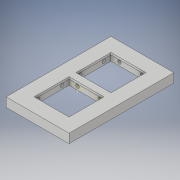
# Autodesk Inventor part: top_plate
Saved by Autodesk Inventor 2018 (Build 220112000, 112)
## iProperties
Created: 2017-12-20
Part Number: top_plate
Material: Generic
Document SubType Name: Modeling
Designer: gaffo
Density: 1 g/cm^3
Appearance: Default
Author: gaffo
Autodesk Inventor part; units mm, degrees
note: some values were not read from the file. Chosen so that the rebuilt part matches the saved one: direction of "Hole6".
ref_plane "YZ Plane" through (0, 0, 0) normal (1, 0, 0) x (0, 1, 0)
ref_plane "XZ Plane" through (0, 0, 0) normal (0, 1, 0) x (-1, 0, 0)
ref_plane "XY Plane" through (0, 0, 0) normal (0, 0, 1) x (1, 0, 0)
sketch "Sketch8" plane through (0, 0, 0) normal (0, 1, 0) x (-1, 0, 0)
  line L0 (45, -75) -> (45, 75) projected
  line L1 (45, 75) -> (-45, 75) projected
  line L2 (-45, 75) -> (-45, -75) projected
  line L3 (-45, -75) -> (45, -75) projected
  line L4 (-27.286, -57.286) -> (-27.286, -2.714) projected
  line L5 (27.286, -57.286) -> (-27.286, -57.286) projected
  line L6 (27.286, -2.714) -> (27.286, -57.286) projected
  line L7 (-27.286, -2.714) -> (27.286, -2.714) projected
  line L8 (27.286, 57.286) -> (27.286, 2.714) projected
  line L9 (27.286, 2.714) -> (-27.286, 2.714) projected
  line L10 (-27.286, 57.286) -> (27.286, 57.286) projected
  line L11 (-27.286, 2.714) -> (-27.286, 57.286) projected
  point P0 (0, 0)
extrude "Extrusion7" add sketch "Sketch8" against normal blind 10
sketch "Sketch2" plane through (0, 0, 0) normal (0, 1, 0) x (-1, 0, 0)
  line L0 (45, 75) -> (-45, 75)
  line L1 (-45, -75) -> (45, -75)
  line L2 (45, -75) -> (45, 75)
  line L3 (-45, 75) -> (-45, -75)
  line L4 (-25, -55) -> (25, -55)
  line L5 (25, -55) -> (25, -5)
  line L6 (25, -5) -> (-25, -5)
  line L7 (-25, -5) -> (-25, -55)
  line L8 (-25, 5) -> (25, 5)
  line L9 (25, 5) -> (25, 55)
  line L10 (25, 55) -> (-25, 55)
  line L11 (-25, 55) -> (-25, 5)
  line L12 (-27.286, 57.286) -> (27.286, 57.286)
  line L13 (27.286, 57.286) -> (27.286, 2.714)
  line L14 (27.286, 2.714) -> (-27.286, 2.714)
  line L15 (-27.286, 2.714) -> (-27.286, 57.286)
  line L16 (-27.286, -2.714) -> (27.286, -2.714)
  line L17 (27.286, -2.714) -> (27.286, -57.286)
  line L18 (27.286, -57.286) -> (-27.286, -57.286)
  line L19 (-27.286, -57.286) -> (-27.286, -2.714)
  point P0 (0, 0)
extrude "Extrusion8" add sketch "Sketch2" along normal blind 3 contours L2 L1 L3 L0 | L12 L13 L14 L15 | L16 L17 L18 L19
hole "Hole1" at (27.286, -5, 12.714) at (27.286, -5, 47.286) at (27.286, -5, -12.714) at (27.286, -5, -47.286) direction (1, 0, 0) diameter 5 depth 5 tip angle 118
hole "Hole2" at (-15.1837, -5, -57.286) at (17.1102, -5, -57.286) direction (0, 0, -1) diameter 5 depth 5 tip angle 118
hole "Hole3" at (-27.286, -5, 47.286) at (-27.286, -5, 12.714) at (-27.286, -5, -12.714) at (-27.286, -5, -47.286) direction (-1, 0, 0) diameter 5 depth 5 tip angle 118
hole "Hole5" at (17.1102, -5, 57.286) at (-15.1837, -5, 57.286) direction (0, 0, 1) diameter 5 depth 5 tip angle 118
hole "Hole6" at (-15.1837, -5, -2.714) at (17.1102, -5, -2.714) direction (0, 0, 1) diameter 5 end up to surface
body "Solid6"
